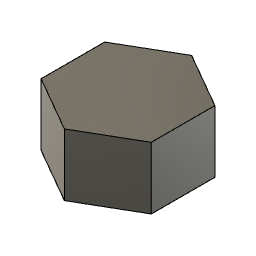
PyPilot_Gehäuse2024 v8 (Autodesk Fusion 360 archive; units mm, degrees)
design "M4-Mutter"
Autodesk Fusion 360 part; units mm, degrees
sketch "Skizze1" plane through (0, 0, 0) normal (0, 1, 0) x (1, 0, 0)
  line L0 (0, 7.7) -> (0, 0)
  line L1 (0, 7.7) -> (0.0094, 3.85)
  line L2 (0, 7.7) -> (0, 0)
  line L3 (-0.0094, -0.25) -> (3.5413, 1.8)
  line L4 (3.5413, 1.8) -> (3.5413, 5.9)
  line L5 (3.5413, 5.9) -> (-0.0095, 7.95)
  line L6 (-0.0095, 7.95) -> (-3.5602, 5.9)
  line L7 (-3.5602, 5.9) -> (-3.5602, 1.8)
  line L8 (-3.5602, 1.8) -> (-0.0094, -0.25)
  point P0 (0.0094, 3.85)
  point P1 (-0.0094, 3.85)
  dimension "d1" = 7.7
  dimension "d3" = 3.85
  dimension "d4" = 7.7
  dimension "d5" = 4.1
  dimension "d6" = 4.1
  dimension "d7" = 4.1
  dimension "d8" = 4.1
  dimension "d9" = 4.1
  dimension "d10" = 4.1
  constraint coincident L0.end L2.end
  constraint vertical L0
  constraint coincident P0 L1.end
  constraint symmetric L1.start L0 L2.start
  constraint symmetric L2.end L0 origin
  measures "d1" distance of L0.start L0.end
  measures "d3" vertical distance of L0.start P0
  measures "d4" distance of L0.start L0.end
  measures "d5" distance of L5.end L6.end
  measures "d6" vertical distance of L6.end L7.end
  measures "d7" vertical distance of L3.end L4.end
  measures "d8" distance of L3.start L3.end
  measures "d9" distance of L3.start L7.end
  measures "d10" distance of L4.end L5.end
extrude "Extrusion1" add sketch "Skizze1" along normal blind 4 makes body 1
copy_body "Körper->Berechn1" bodies 1 removing the originals makes body 2 in component "Component"
component "Component" placed x (1, 0, 0) y (0, 1, 0) z (0, 0, 1) at (0, 0, 0)
